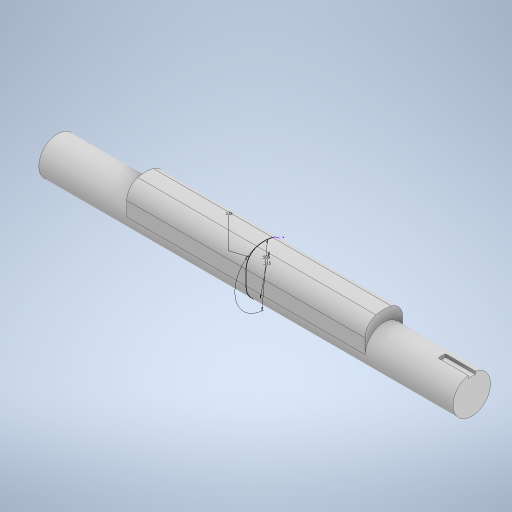
# Autodesk Inventor part: Cam Shaft Test
Saved by Autodesk Inventor 2023 (Build 270158000, 158)
## iProperties
Created: 2022-12-25
Part Number: Cam Shaft Test
Material: Generic
Document SubType Name: Modeling
Designer: tgr41
Density: 1 g/cm^3
Appearance: Default
Author: tgr41
Autodesk Inventor part; units mm, degrees
ref_plane "YZ Plane" through (0, 0, 0) normal (1, 0, 0) x (0, 1, 0)
ref_plane "XZ Plane" through (0, 0, 0) normal (0, 1, 0) x (-1, 0, 0)
ref_plane "XY Plane" through (0, 0, 0) normal (0, 0, 1) x (1, 0, 0)
sketch "Sketch1" plane through (0, 0, 0) normal (1, 0, 0) x (0, 1, 0)
  circle A0 centre (0, 0) radius 4
  arc A1 (6.1319, -1.65) -> (6.1319, 1.65) centre (0, 0) ccw
  line L0 (0, 4) -> (3.0659, 4)
  line L1 (0, -4) -> (3.0659, -4)
  arc A2 (6.1319, 1.65) -> (3.0659, 4) centre (3.0659, 0.825) ccw
  arc A3 (3.0659, -4) -> (6.1319, -1.65) centre (3.0659, -0.825) ccw
  point P0 (4.9318, 4)
  point P1 (4.9318, -4)
  dimension "d0" = 8
  dimension "d1" = 12.7
  dimension "d2" = 3.175
  constraints: 10 point on circle, 5 tangent, 4 centre point, 4 end point, 2 coincident, 2 point on line, 1 equal radius, 1 horizontal, 1 parallel
  measures "d0" diameter of A0
  measures "d1" diameter of A1
  measures "d2" radius of A2
extrude "Extrusion1" add sketch "Sketch1" along normal mid plane 88.2904 contours A0
extrude "Extrusion2" add sketch "Sketch1" along normal mid plane 50.8 contours A0 L0 A2 A1 A3 L1
sketch "Sketch2" plane through (44.1452, 0, 0) normal (1, 0, 0) x (0, 0, -1)
  circle A0 centre (0, 0) radius 4 projected
  line L0 (0, 0) -> (0, 3.3434)
  line L1 (0, 3.3434) -> (0.7706, 3.3434)
  line L2 (0.7706, 3.3434) -> (0.7706, 3.9251)
  line L3 (0, 3.3434) -> (-0.7706, 3.3434)
  line L4 (-0.7706, 3.3434) -> (-0.7706, 3.9251)
  constraints: 10 end point, 2 perpendicular, 2 symmetric about line, 1 vertical, 2 other
extrude "Extrusion3" cut sketch "Sketch2" against normal blind 6.35 contours L2 L1 L3 L4 A0 picked at (0.343, 3.5595)
body "Solid1"
